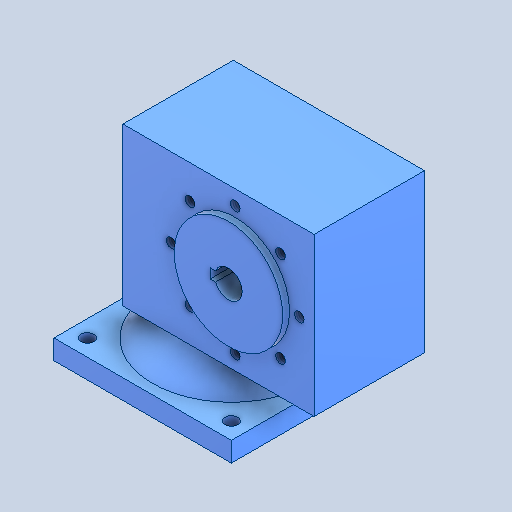
# Autodesk Inventor part: motor_gear_head
Saved by Autodesk Inventor 2025.3 (Build 293356030, 356C)
## iProperties
Created: 2025-08-25
Part Number: motor_gear_head
Material: ABS 플라스틱
Document SubType Name: Modeling
Designer: MSI
Density: 1.06 g/cm^3
Appearance: 매끄러움 - 흰색
Mass: 598.544 g
Surface Area: 611.158 cm^2
Volume: 564.664 cm^3
Author: MSI
Autodesk Inventor part; units mm, degrees
ref_plane "YZ Plane" through (0, 0, 0) normal (1, 0, 0) x (0, 1, 0)
ref_plane "XZ Plane" through (0, 0, 0) normal (0, 1, 0) x (-1, 0, 0)
ref_plane "XY Plane" through (0, 0, 0) normal (0, 0, 1) x (1, 0, 0)
sketch "스케치1" plane through (0, 0, 0) normal (0, 1, 0) x (-1, 0, 0)
  line L0 (45, 45) -> (-45, 45)
  line L1 (-45, 45) -> (-45, -45)
  line L2 (-45, -45) -> (45, -45)
  line L3 (45, -45) -> (45, 45)
  line L4 (45, 45) -> (-45, -45) construction
  line L5 (-45, 45) -> (45, -45) construction
  point P0 (0, 0)
  dimension "d0" = 90
  dimension "d1" = 90
  constraints: 12 end point, 2 midpoint, 2 parallel, 1 horizontal, 1 perpendicular
  measures "d0" distance of L2.end L1.end
  measures "d1" distance of L1.end L0.end
extrude "돌출1" add sketch "스케치1" along normal blind 10
sketch "스케치2" plane through (0, 10, 0) normal (0, 1, 0) x (1, 0, 0)
  circle A0 centre (0, 0) radius 40
  dimension "d4" = 80
  constraints: 1 centre point, 1 coincident
  measures "d4" diameter of A0
extrude "돌출2" add sketch "스케치2" along normal blind 14.5
draft "면 구배1" angle 45 pull direction (0, 1, 0) fixed plane through (-43.2552, 10, 1.4416) normal (0, 1, 0) faces at (-36.8857, 19.6667, -15.474)
sketch "스케치3" plane through (0, 24.5, 0) normal (0, 1, 0) x (1, 0, 0)
  line L0 (-27, 28) -> (70, 28)
  line L1 (70, 28) -> (70, -28)
  line L2 (70, -28) -> (-27, -28)
  line L3 (-27, -28) -> (-27, 28)
  line L4 (30, -28) -> (30, 28) construction
  point P0 (0, 0)
  point P1 (-27, 0)
  dimension "d8" = 56
  dimension "d9" = 30
  dimension "d10" = 57
  dimension "d11" = 40
  constraints: 10 end point, 2 parallel, 2 perpendicular, 2 point on line, 1 horizontal, 1 horizontal alignment, 1 midpoint
  measures "d8" distance of L2.end L0.start
  measures "d9" distance from line of L4 point (0, 0)
  measures "d10" distance between parallel lines of L4 L3
  measures "d11" distance between parallel lines of L1 L4
extrude "돌출3" add sketch "스케치3" along normal blind 80
sketch "스케치4" plane through (0, 0, 0) normal (0, 0, 1) x (1, 0, 0)
  circle A0 centre (30, 64.5) radius 27.5
  line L0 (-27, 24.5) -> (-27, 104.5) projected
  point P0 (0, 0)
  point P1 (-27, 64.5)
  dimension "d14" = 55
  dimension "d15" = 57
  constraints: 1 centre point, 1 horizontal alignment, 1 midpoint
  measures "d14" diameter of A0
  measures "d15" distance from line of A0.centre L0
extrude "돌출4" add sketch "스케치4" along normal mid plane 63
sketch "스케치5" plane through (30, 64.5, 31.5) normal (0, 0, 1) x (1, 0, 0)
  circle A0 centre (0, 0) radius 27.5 projected
  circle A1 centre (0, 0) radius 7
  line L0 (-4.7, 2.5) -> (-9.3, 2.5)
  line L1 (-9.3, 2.5) -> (-9.3, -2.5)
  line L2 (-9.3, -2.5) -> (-4.7, -2.5)
  line L3 (-4.7, -2.5) -> (-4.7, 2.5)
  line L4 (-4.7, 2.5) -> (-9.3, -2.5) construction
  line L5 (-9.3, 2.5) -> (-4.7, -2.5) construction
  point P0 (-30, -64.5)
  point P1 (-7, 0)
  point P2 (-6.5383, -2.5)
  point P3 (-6.5383, 2.5)
  dimension "d18" = 14
  dimension "d19" = 5
  dimension "d20" = 16.3
  constraints: 12 end point, 2 midpoint, 2 parallel, 1 coincident, 1 horizontal, 1 horizontal alignment, 1 perpendicular, 3 other
  measures "d19" distance of L0.end L1.end
extrude "돌출5" cut sketch "스케치5" against normal through all contours A1 L2 L3 L0 | L0 L3 L2 A1 | A1 L2 L1 L0
sketch "스케치6" plane through (-27, 24.5, 28) normal (0, 0, 1) x (1, 0, 0)
  circle A0 centre (57, 40) radius 27.5 projected
  line L0 (57, 40) -> (57, 72.5) construction
  point P0 (27, -24.5)
  dimension "d23" = 32.5
  constraints: 2 end point, 1 vertical
  measures "d23" distance of L0.start L0.end
hole "구멍1" at (30, 97, 28) direction (0, 0, -1) diameter 4.917 depth 17.1 tip angle 118 thread size "M6x1" class "6H" standard "ISO Metric profile"
pattern_circular "원형 패턴1" count 8 over 360 about axis through (30, 64.5, 0) along (0, 0, 1) of "구멍1"
mirror "미러1" about plane through (0, 0, 0) normal (0, 0, 1) of "구멍1", "원형 패턴1"
sketch "스케치7" plane through (0, 10, 0) normal (0, 1, 0) x (1, 0, 0)
  line L0 (36.5, 36.5) -> (-36.5, 36.5) construction
  line L1 (-36.5, 36.5) -> (-36.5, -36.5) construction
  line L2 (-36.5, -36.5) -> (36.5, -36.5) construction
  line L3 (36.5, -36.5) -> (36.5, 36.5) construction
  line L4 (36.5, 36.5) -> (-36.5, -36.5) construction
  line L5 (-36.5, 36.5) -> (36.5, -36.5) construction
  point P0 (0, 0)
  dimension "d34" = 73
  dimension "d35" = 73
  constraints: 12 end point, 2 midpoint, 2 parallel, 1 horizontal, 1 perpendicular
  measures "d34" distance of L2.end L1.end
  measures "d35" distance of L1.end L0.end
hole "구멍2" at (-36.5, 10, 36.5) at (36.5, 10, 36.5) at (-36.5, 10, -36.5) at (36.5, 10, -36.5) direction (0, -1, 0) diameter 6.6 end through all clearance for "Countersunk Flat Head Screw ISO 2009/7046" size "M6" standard "ISO"
